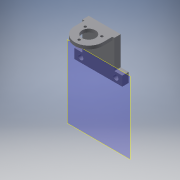
# Autodesk Inventor part: encoder bracket
Saved by Autodesk Inventor 2016 (Build 200138000, 138)
## iProperties
Created: 2017-06-15
Part Number: encoder bracket
Material: Generic
Document SubType Name: Modeling
Designer: RMcComber
Density: 1 g/cm^3
Appearance: Default
Author: RMcComber
Autodesk Inventor part; units mm, degrees
ref_plane "YZ Plane" through (0, 0, 0) normal (1, 0, 0) x (0, 1, 0)
ref_plane "XZ Plane" through (0, 0, 0) normal (0, 1, 0) x (-1, 0, 0)
ref_plane "XY Plane" through (0, 0, 0) normal (0, 0, 1) x (1, 0, 0)
ref_plane "Work Plane1" through (45.4774, 14.9992, -51) normal (0, 1, 0) x (0, 0, -1)
sketch "Sketch1" plane through (45.4774, 14.9992, -51) normal (0, 1, 0) x (0, 0, -1)
  line L0 (-43.5, 30.4092) -> (-43.5, -29.5908) construction
  line L1 (-36, 37.9092) -> (-51, 37.9092)
  line L2 (-51, 37.9092) -> (-51, -37.0908)
  line L3 (-51, -37.0908) -> (-36, -37.0908)
  line L4 (-36, -37.0908) -> (-36, 37.9092)
  circle A0 centre (-43.5, 30.4092) radius 4
  circle A1 centre (-43.5, -29.5908) radius 4
  line L5 (-51, 25.4092) -> (-91, 25.4092)
  line L6 (-91, 25.4092) -> (-91, -24.5908)
  line L7 (-91, -24.5908) -> (-51, -24.5908)
  line L8 (-51, -24.5908) -> (-51, 25.4092)
  circle A2 centre (93.5, 21.4092) radius 4 projected
  circle A3 centre (93.5, -20.5908) radius 4 projected
  line L9 (51, -30.5908) -> (51, 31.4092) projected
  line L10 (51, 31.4092) -> (86, 31.4092) projected
  line L11 (86, 31.4092) -> (86, -30.5908) projected
  line L12 (86, -30.5908) -> (51, -30.5908) projected
  circle A4 centre (-43.5, 30.4092) radius 4 projected
  circle A5 centre (43.5, -29.5908) radius 4 projected
  circle A6 centre (0, -29.5908) radius 4 projected
  circle A7 centre (0, 30.4092) radius 4 projected
  circle A8 centre (43.5, 30.4092) radius 4 projected
  circle A9 centre (-43.5, -29.5908) radius 4 projected
  line L13 (-36, -34.5908) -> (-36, 35.4092) projected
  line L14 (-36, 35.4092) -> (-8, 35.4092) projected
  line L15 (-8, 35.4092) -> (-8, -34.5908) projected
  line L16 (-8, -34.5908) -> (-36, -34.5908) projected
  line L17 (8, -34.5908) -> (8, 35.4092) projected
  line L18 (8, 35.4092) -> (36, 35.4092) projected
  line L19 (36, 35.4092) -> (36, -34.5908) projected
  line L20 (36, -34.5908) -> (8, -34.5908) projected
  line L21 (-51, -44.5908) -> (101, -44.5908) projected
  line L22 (101, -44.5908) -> (101, 45.4092) projected
  line L23 (101, 45.4092) -> (-51, 45.4092) projected
  line L24 (-51, 45.4092) -> (-51, -44.5908) projected
  point P0 (-51, 0.4092)
  point P1 (-36, 0.4092)
  dimension "d0" = 75
  dimension "d1" = 15
  dimension "d2" = 40
  dimension "d3" = 50
  dimension "d14" = 8
  constraints: 18 end point, 4 coincident, 4 midpoint, 4 parallel, 2 centre point, 2 horizontal, 2 perpendicular, 1 equal radius
  measures "d0" distance of L1.end L2.end
  measures "d1" distance of L1.start L1.end
  measures "d2" distance of L5.start L5.end
  measures "d3" distance of L5.end L6.end
  measures "d14" diameter of A1
extrude "Extrusion1" add sketch "Sketch1" along normal blind 10 contours L4 L3 L2 L1 | L2 L7 L6 L5
sketch "Sketch2" plane through (20.0682, 14.9992, 40) normal (0, 0, 1) x (1, 0, 0)
  line L0 (0, 0) -> (50, 0) projected
  line L1 (50, 0) -> (50, 10) projected
  line L2 (0, 10) -> (50, 10) projected
  line L3 (0, 0) -> (0, 10) projected
  arc A0 (36, -15) -> (14, -15) centre (25, -15) ccw construction
  arc A1 (3, -15) -> (47, -15) centre (25, -15) ccw
  line L4 (3, -15) -> (3, 0)
  line L5 (47, -15) -> (47, 0)
  circle A2 centre (25, -15) radius 10.5
  circle A3 centre (25, -15) radius 15 construction
  circle A4 centre (25, -30) radius 2
  circle A5 centre (12.0096, -7.5) radius 2
  circle A6 centre (37.9904, -7.5) radius 2
  line L6 (25, -15) -> (25, -30) construction
  line L7 (25, -15) -> (37.9904, -7.5) construction
  line L8 (25, -15) -> (12.0096, -7.5) construction
  point P0 (-20.0682, -14.9992)
  dimension "d6" = 22
  dimension "d7" = 21
  dimension "d8" = 30
  dimension "d9" = 4
  dimension "d10" = 120
  dimension "d11" = 120
  constraints: 10 end point, 6 centre point, 5 point on circle, 3 coincident, 2 equal radius, 2 perpendicular, 2 point on line, 2 tangent, 1 parallel
  measures "d6" radius of A1
  measures "d7" diameter of A2
  measures "d8" diameter of A3
  measures "d9" diameter of A4
  measures "d10" angle of L6 L8
  measures "d11" angle of L6 L7
extrude "Extrusion2" add sketch "Sketch2" along normal blind 5
body "Solid1"
